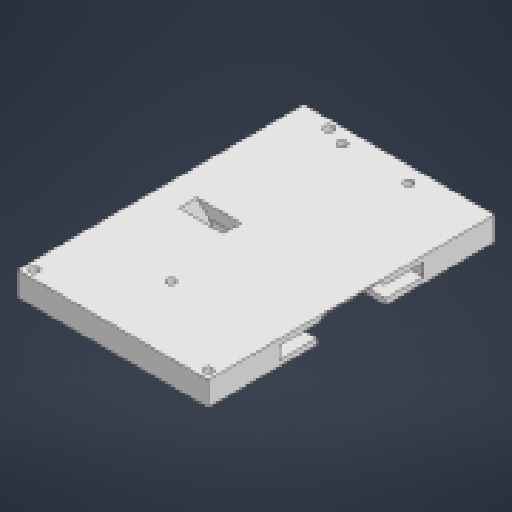
# Autodesk Inventor part: PCB_Housing_01_V4
Saved by Autodesk Inventor 2026.2 (Build 302298000, 298)
## iProperties
Created: 2026-03-15
Part Number: PCB_Housing_01_V4
Material: Generic
Document SubType Name: Modeling
Designer: vckot
Density: 1 g/cm^3
Appearance: Default
Author: vckot
Autodesk Inventor part; units mm, degrees
ref_plane "YZ Plane" through (0, 0, 0) normal (1, 0, 0) x (0, 1, 0)
ref_plane "XZ Plane" through (0, 0, 0) normal (0, 1, 0) x (-1, 0, 0)
ref_plane "XY Plane" through (0, 0, 0) normal (0, 0, 1) x (1, 0, 0)
sketch "Sketch1" plane through (0, 0, 0) normal (0, 1, 0) x (-1, 0, 0)
  line L0 (40, 60) -> (-40, 60)
  line L1 (-40, 60) -> (-40, -60)
  line L2 (-40, -60) -> (40, -60)
  line L3 (40, -60) -> (40, 60)
  line L4 (40, 60) -> (-40, -60) construction
  line L5 (-40, 60) -> (40, -60) construction
  point P0 (0, 0)
  dimension "d0" = 80
  dimension "d1" = 120
  constraints: 12 end point, 2 midpoint, 2 parallel, 1 horizontal, 1 perpendicular
  measures "d0" distance of L2.end L1.end
  measures "d1" distance of L1.end L0.end
extrude "Extrusion1" add sketch "Sketch1" along normal mid plane 10
sketch "Sketch3" plane through (0, -5, 0) normal (0, -1, 0) x (1, 0, 0)
  circle A0 centre (-36.5, 56.5) radius 2.25 projected
  circle A1 centre (36.5, 56.5) radius 2.25 projected
  circle A2 centre (-26, -56.5) radius 2.25 projected
  circle A3 centre (-17.5, -53.5) radius 2.25 projected
  circle A4 centre (10.5, -53.5) radius 2.25 projected
  circle A5 centre (-3.5, 32) radius 2.25 projected
  point P0 (0, 0)
hole "Hole1" at (-36.5, -5, 56.5) at (36.5, -5, 56.5) at (-26, -5, -56.5) at (-17.5, -5, -53.5) at (10.5, -5, -53.5) at (-3.5, -5, 32) direction (0, 1, 0) diameter 3.75 end through all counterbore diameter 6 counterbore depth 3.5
sketch "Sketch4" plane through (40, -5, -60) normal (1, 0, 0) x (0, 0, -1)
  circle A0 centre (-60, 5) radius 4.125
  line L0 (-64.125, 5) -> (-64.125, 0)
  line L1 (-120, 0) -> (0, 0) projected
  line L2 (-55.875, 5) -> (-55.875, 0)
  line L3 (-64.125, 0) -> (-55.875, 0)
  circle A1 centre (-70, 5) radius 2.25
  circle A2 centre (-50, 5) radius 2.25
  arc A3 (-70, 9.125) -> (-74.125, 5) centre (-70, 5) ccw
  arc A4 (-45.875, 5) -> (-50, 9.125) centre (-50, 5) ccw
  line L4 (-70, 9.125) -> (-60, 9.125)
  line L5 (-50, 9.125) -> (-60, 9.125)
  line L6 (-74.125, 5) -> (-74.125, 0)
  line L7 (-45.875, 5) -> (-45.875, 0)
  line L8 (-74.125, 0) -> (-45.875, 0)
  line L9 (-120, 10) -> (-120, 0) projected
  line L10 (0, 0) -> (0, 10) projected
  circle A5 centre (-60, 5) radius 2.625
  point P0 (-120, 5)
  point P1 (0, 5)
  dimension "d21" = 8.25
  dimension "d22" = 4.5
  dimension "d23" = 4.5
  dimension "d24" = 10
  dimension "d26" = 10
  dimension "d27" = 8.25
  dimension "d28" = 8.25
  dimension "d35" = 5.25
  constraints: 16 end point, 8 point on circle, 6 centre point, 6 point on line, 5 tangent, 4 coincident, 4 perpendicular, 2 horizontal alignment, 2 midpoint, 1 horizontal, 1 parallel, 1 vertical
  measures "d21" diameter of A0
  measures "d22" diameter of A1
  measures "d23" diameter of A2
  measures "d24" distance of A0.centre A1.centre
  measures "d26" distance of A0.centre A2.centre
  measures "d27" diameter of A3
  measures "d28" diameter of A4
  measures "d35" diameter of A5
extrude "Extrusion4" cut sketch "Sketch4" against normal blind 40 contours A0 | L2 L1 L0 A0 | A0 L5 A4 L7 L1 L2 | A0 L0 L1 L6 A3 L4 | A5
extrude "Extrusion5" cut sketch "Sketch4" against normal blind 48 contours A1 | A2
thicken "Thicken1" operation add thickness 0.25 both sides no extend neighbours yes toward (0, 1, 0) faces at (26.6667, 4.125, -3.3333) (13.3333, 3.4082, 12.3237) (13.3333, -1.6667, 14.125) (13.3333, 4.1135, -10.3083) (13.3333, -3.3333, -14.125)
extrude "Extrusion6" cut sketch "Sketch4" against normal blind 60 contours A5
sketch "Sketch5" plane through (-20, 0, 0) normal (1, 0, 0) x (0, 0, -1)
  circle A0 centre (0, 0) radius 3.75
  dimension "d38" = 7.5
  constraints: 1 centre point, 1 coincident
  measures "d38" diameter of A0
extrude "Extrusion7" cut sketch "Sketch5" along normal blind 10
sketch "Sketch6" plane through (0, 5, 0) normal (0, 1, 0) x (1, 0, 0)
  line L0 (-20, 3.75) -> (-10, 3.75) projected
  line L1 (-20, -3.75) -> (-20, 3.75) projected
  line L2 (-20, -3.75) -> (-10, -3.75) projected
  line L3 (-10, -3.75) -> (-10, 3.75) projected
  point P0 (0, 0)
extrude "Extrusion8" cut sketch "Sketch6" against normal blind 5
chamfer "Chamfer1" distance 8.5 angle 45 1 edges at (-20, 5, 0)
sketch "Sketch7" plane through (40, -5, -60) normal (1, 0, 0) x (0, 0, -1)
  line L0 (-87.5, 2.5) -> (-32.5, 2.5)
  line L1 (-32.5, 2.5) -> (-32.5, 7.5)
  line L2 (-32.5, 7.5) -> (-87.5, 7.5)
  line L3 (-87.5, 7.5) -> (-87.5, 2.5)
  line L4 (-87.5, 2.5) -> (-32.5, 7.5) construction
  line L5 (-32.5, 2.5) -> (-87.5, 7.5) construction
  line L6 (-87.625, 2.375) -> (-32.375, 2.375)
  line L7 (-32.375, 2.375) -> (-32.375, 7.625)
  line L8 (-32.375, 7.625) -> (-87.625, 7.625)
  line L9 (-87.625, 7.625) -> (-87.625, 2.375)
  point P0 (-60, 5)
  dimension "d46" = 55
  dimension "d47" = 5
  dimension "d48" = 0.125
  constraints: 20 end point, 4 parallel, 2 midpoint, 2 perpendicular, 1 horizontal, 3 other
  measures "d46" distance of L2.end L1.end
  measures "d47" distance of L1.end L0.end
  measures "d48" distance between parallel lines of L3 L9
extrude "Extrusion9" cut sketch "Sketch7" against normal blind 36 contours L3 L2 L1 L0 | L9 L8 L7 L6
equation "\"d27\" = d21"
equation "\"d28\" = d21"
body "Solid1"
